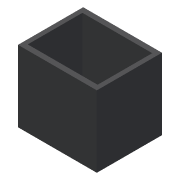
# Autodesk Inventor part: 17-0028-0033
Saved by Autodesk Inventor 2016 SP2 (Build 200236200, 236)
## iProperties
Category: IOP
Company: Universiteit van Amsterdam
Created: 2017-11-20
Part Number: 17-0028-0033
Material: Steel, constructie staal
Document SubType Name: Modeling
Designer: Daan Giesen
Density: 7.85 g/cm^3
Appearance: Gray
Project: Digital PID Loop
Cost Center: 17-0028
User Status: Work in Progress
Authority: Reichsöllner, Lukas
Author: Daan Giesen
Title: Digital PID Loop
Revision Number: A
Autodesk Inventor part; units mm, degrees
ref_plane "YZ Plane" through (0, 0, 0) normal (1, 0, 0) x (0, 1, 0)
ref_plane "XZ Plane" through (0, 0, 0) normal (0, 1, 0) x (-1, 0, 0)
ref_plane "XY Plane" through (0, 0, 0) normal (0, 0, 1) x (1, 0, 0)
sketch "Sketch1" plane through (0, 0, 0) normal (0, 0, 1) x (1, 0, 0)
  line L0 (0, 294) -> (0, -294) construction
  line L1 (-355.6, 0) -> (355.6, 0) construction
  line L2 (254, -210) -> (-254, -210)
  line L3 (-254, -210) -> (-254, 210)
  line L4 (-254, 210) -> (254, 210)
  line L5 (254, 210) -> (254, -210)
  line L6 (254, -210) -> (-254, 210) construction
  line L7 (-254, -210) -> (254, 210) construction
  point P0 (0, 0)
  dimension "d4" = 420
  dimension "d5" = 508
  constraints: 12 end point, 2 midpoint, 2 parallel, 1 horizontal, 1 perpendicular
  measures "d4" distance of L2.end L3.end
  measures "d5" distance of L3.end L4.end
extrude "Extrusion3" add sketch "Sketch1" along normal mid plane 459.994
sketch "Sketch2" plane through (0, 0, 229.997) normal (0, 0, 1) x (1, 0, 0)
  line L0 (225, -176) -> (-225, -176)
  line L1 (-225, -176) -> (-225, 176)
  line L2 (-225, 176) -> (225, 176)
  line L3 (225, 176) -> (225, -176)
  line L4 (225, -176) -> (-225, 176) construction
  line L5 (-225, -176) -> (225, 176) construction
  point P0 (0, 0)
  dimension "d8" = 450
  dimension "d9" = 352
  constraints: 12 end point, 2 midpoint, 2 parallel, 1 horizontal, 1 perpendicular
  measures "d8" distance of L1.end L2.end
  measures "d9" distance of L0.end L1.end
extrude "Extrusion4" cut sketch "Sketch2" against normal through all
body "Solid3"
